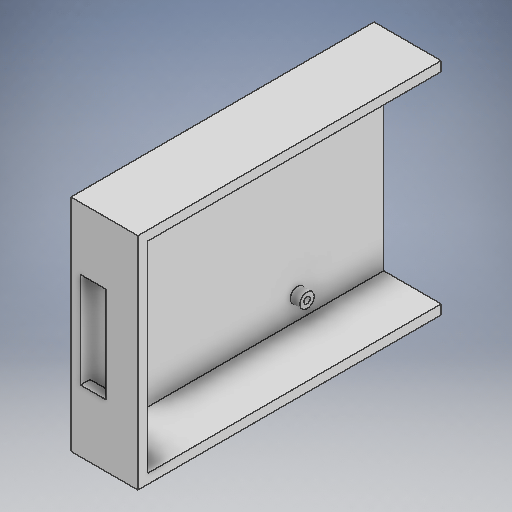
# Autodesk Inventor part: RP5_case
Saved by Autodesk Inventor 2026.1 (Build 301233000, 233)
## iProperties
Created: 2025-12-08
Part Number: RP5_case
Material: Generic
Document SubType Name: Modeling
Designer: emanuel
Density: 1 g/cm^3
Appearance: Default
Author: emanuel
Autodesk Inventor part; units mm, degrees
ref_plane "YZ Plane" through (0, 0, 0) normal (1, 0, 0) x (0, 1, 0)
ref_plane "XZ Plane" through (0, 0, 0) normal (0, 1, 0) x (-1, 0, 0)
ref_plane "XY Plane" through (0, 0, 0) normal (0, 0, 1) x (1, 0, 0)
sketch "Sketch1" plane through (0, 0, 0) normal (1, 0, 0) x (0, 1, 0)
  line L0 (0, 0) -> (49, 0)
  line L1 (49, 0) -> (49, -58)
  line L2 (49, -58) -> (0, -58)
  line L3 (0, -58) -> (0, 0)
  circle A0 centre (49, 0) radius 1
  circle A1 centre (49, -58) radius 1
  circle A2 centre (0, -58) radius 1
  circle A3 centre (0, 0) radius 1
  line L4 (49, 0) -> (49, 7)
  line L5 (49, 7) -> (56, 7)
  line L6 (0, 0) -> (-7, 0)
  line L7 (56, 7) -> (56, -85)
  line L8 (56, 7) -> (-7, 7)
  line L9 (-7, 7) -> (-7, -85)
  line L10 (-7, -85) -> (56, -85)
  line L11 (56, -85) -> (56, 7)
  line L12 (49, 0) -> (52.5, 0)
  line L13 (52.5, 0) -> (52.5, 3.5)
  line L14 (52.5, 3.5) -> (49, 3.5)
  line L15 (49, 3.5) -> (49, 0)
  line L16 (52.5, 3.5) -> (-3.5, 3.5)
  line L17 (-3.5, 3.5) -> (-3.5, -81.5)
  line L18 (-3.5, -81.5) -> (52.5, -81.5)
  line L19 (52.5, -81.5) -> (52.5, 3.5)
  line L20 (56, 7) -> (59, 7)
  line L21 (59, 7) -> (59, 10)
  line L22 (59, 10) -> (56, 10)
  line L23 (56, 10) -> (56, 7)
  line L24 (-7, -85) -> (-10, -85)
  line L25 (-10, -85) -> (-10, -82)
  line L26 (-10, -82) -> (-7, -82)
  line L27 (-7, -82) -> (-7, -85)
  line L28 (59, 10) -> (-10, 10)
  line L29 (-10, 10) -> (-10, -85)
  line L30 (-10, -85) -> (59, -85)
  line L31 (59, -85) -> (59, 10)
  dimension "d0" = 49
  dimension "d1" = 58
  dimension "d2" = 2
  dimension "d3" = 2
  dimension "d4" = 2
  dimension "d5" = 2
  dimension "d6" = 7
  dimension "d7" = 7
  dimension "d8" = 7
  dimension "d9" = 92
  dimension "d10" = 3.5
  dimension "d11" = 3.5
  dimension "d12" = 56
  dimension "d13" = 85
  dimension "d14" = 3
  dimension "d15" = 3
  dimension "d16" = 3
  dimension "d17" = 3
  constraints: 64 end point, 14 parallel, 8 horizontal, 7 perpendicular, 4 centre point, 4 coincident, 2 vertical, 1 point on line
  measures "d0" distance of L1.end L2.end
  measures "d1" distance of L0.end L1.end
  measures "d2" diameter of A0
  measures "d3" diameter of A1
  measures "d4" diameter of A2
  measures "d5" diameter of A3
  measures "d6" distance of L4.start L4.end
  measures "d7" distance of L4.end L5.end
  measures "d8" distance of L6.start L6.end
  measures "d9" distance of L5.end L7.end
  measures "d10" distance of L14.end L13.end
  measures "d11" distance of L13.end L12.end
  measures "d12" distance of L18.end L17.end
  measures "d13" distance of L17.end L16.end
  measures "d14" distance of L22.end L21.end
  measures "d15" distance of L21.end L20.end
  measures "d16" distance of L25.end L26.end
  measures "d17" distance of L24.end L25.end
extrude "Extrusion1" add sketch "Sketch1" along normal blind 3 contours A3 L6 L17 L16 L4 A0 L0 | L0 A0 L1 A1 L2 A2 L3 A3 | L3 A2 L2 A1 L1 A0 L12 L19 L18 L17 L6 A3 | L17 L18 L19 L13 L14 L4 L5 L7 L10 L9 L6 | L6 L9 L8 L4 L16 L17 | L4 L14 L13 L12 A0 | L9 L26 L29 L28 L23 L5 L8 | L9 L24 L25 L26 | L20 L31 L30 L7 | L23 L22 L21 L20
sketch "Sketch2" plane through (3, 0, 0) normal (1, 0, 0) x (0, 0, -1)
  circle A0 centre (0, 49) radius 1 projected
  circle A1 centre (0, 49) radius 2.25
  circle A2 centre (58, 49) radius 1 projected
  circle A3 centre (58, 49) radius 2.25
  circle A4 centre (0, 0) radius 1 projected
  circle A5 centre (0, 0) radius 2.25
  circle A6 centre (58, 0) radius 1 projected
  circle A7 centre (58, 0) radius 2.25
  circle A8 centre (0, 49) radius 1
  circle A9 centre (58, 49) radius 1
  circle A10 centre (0, 0) radius 1
  circle A11 centre (58, 0) radius 1
  line L0 (85, 59) -> (-10, 59) projected
  line L1 (-10, 59) -> (-7, 59)
  line L2 (-7, 59) -> (-7, 56)
  line L3 (-7, 56) -> (-10, 56)
  line L4 (-10, 56) -> (-10, 59)
  line L5 (-10, -10) -> (85, -10) projected
  line L6 (85, -10) -> (82, -10)
  line L7 (82, -10) -> (82, -7)
  line L8 (82, -7) -> (85, -7)
  line L9 (85, -7) -> (85, -10)
  line L10 (-7, 56) -> (82, 56)
  line L11 (82, 56) -> (82, -7)
  line L12 (82, -7) -> (-7, -7)
  line L13 (-7, -7) -> (-7, 56)
  line L14 (-10, 59) -> (-10, -10)
  line L15 (-10, 59) -> (-10, -10) projected
  line L16 (-10, 24.5) -> (-7, 24.5)
  line L17 (-18.5, 39.5) -> (1.5, 39.5)
  line L18 (1.5, 39.5) -> (1.5, 9.5)
  line L19 (1.5, 9.5) -> (-18.5, 9.5)
  line L20 (-18.5, 9.5) -> (-18.5, 39.5)
  line L21 (-18.5, 39.5) -> (1.5, 9.5) construction
  line L22 (1.5, 39.5) -> (-18.5, 9.5) construction
  line L23 (-10, 59) -> (85, 59)
  line L24 (85, 59) -> (85, -10)
  line L25 (85, -10) -> (-10, -10)
  line L26 (-10, -10) -> (-10, 59)
  line L27 (82, 56) -> (85, 56)
  point P0 (-8.5, 24.5)
  point P1 (-7, 9.5)
  point P2 (-10, 9.5)
  point P3 (-10, 39.5)
  point P4 (-7, 39.5)
  dimension "d20" = 4.5
  dimension "d21" = 4.5
  dimension "d22" = 4.5
  dimension "d23" = 4.5
  dimension "d24" = 3
  dimension "d25" = 3
  dimension "d26" = 3
  dimension "d27" = 3
  dimension "d28" = 20
  dimension "d29" = 30
  constraints: 50 end point, 10 parallel, 8 centre point, 8 coincident, 6 perpendicular, 5 horizontal, 5 midpoint, 1 concentric, 1 point on line, 1 vertical
  measures "d20" diameter of A1
  measures "d21" diameter of A3
  measures "d22" diameter of A5
  measures "d23" diameter of A7
  measures "d24" distance of L2.end L3.end
  measures "d25" distance of L1.end L2.end
  measures "d26" distance of L7.end L8.end
  measures "d27" distance of L6.end L7.end
  measures "d28" distance of L18.end L19.end
  measures "d29" distance of L17.end L18.end
extrude "Extrusion2" add sketch "Sketch2" along normal blind 8 contours L24 L27 L10 L2 L0 | L2 L3 L4 L0 | L13 L17 L14 L3 | L9 L5 L7 L8 | L7 L5 L14 L19 L13 L12
extrude "Extrusion3" add sketch "Sketch2" along normal blind 3 contours A1 | A3 | A5 | A7
sketch "Sketch3" plane through (11, 0, 0) normal (1, 0, 0) x (0, 0, -1)
  line L0 (85, 59) -> (-10, 59) projected
  line L1 (85, -10) -> (85, 59) projected
  line L2 (-10, 59) -> (85, 59)
  line L3 (85, 59) -> (85, -10)
  line L4 (85, -10) -> (-10, -10)
  line L5 (-10, -10) -> (-10, 59)
  line L6 (85, 56) -> (-7, 56) projected
  line L7 (-7, -7) -> (85, -7) projected
  line L8 (-7, 56) -> (85, 56)
  line L9 (85, 56) -> (85, -7)
  line L10 (85, -7) -> (-7, -7)
  line L11 (-7, -7) -> (-7, 56)
  point P0 (0, 0)
  constraints: 16 end point, 4 parallel, 2 horizontal, 2 perpendicular
extrude "Extrusion4" add sketch "Sketch3" along normal blind 10 contours L1 L6 L11 L7 L4 L5 L0
body "Solid1"
